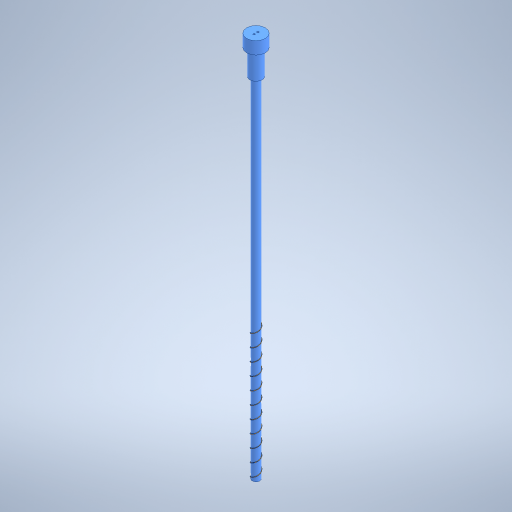
# Autodesk Inventor part: heater plug
Saved by Autodesk Inventor 2023 (Build 270158030, 158C)
## iProperties
Created: 2025-06-04
Part Number: heater plug
Material: Generisch
Document SubType Name: Modeling
Designer: Julian
Density: 1 g/cm^3
Appearance: Vorgabe
Author: Julian
Autodesk Inventor part; units mm, degrees
ref_plane "YZ Plane" through (0, 0, 0) normal (1, 0, 0) x (0, 1, 0)
ref_plane "XZ Plane" through (0, 0, 0) normal (0, 1, 0) x (-1, 0, 0)
sketch "Skizze1" plane through (0, 0, 0) normal (0, 1, 0) x (-1, 0, 0)
  circle A0 centre (0, 0) radius 7.5
  circle A1 centre (0, 0) radius 5
  circle A2 centre (0, 0) radius 3
  line L0 (0, 5) -> (0, 1.5)
  line L1 (0, 1.5) -> (0, -1.5)
  circle A3 centre (0, -1.5) radius 0.75
  circle A4 centre (0, 1.5) radius 0.75
  dimension "d1" = 10
  dimension "d0" = 15
  dimension "d2" = 6
  dimension "d3" = 3.5
  dimension "d4" = 3
  dimension "d5" = 1.5
  dimension "d6" = 1.5
  constraints: 5 coincident, 4 centre point, 4 end point, 1 point on line, 1 vertical, 1 vertical alignment, 2 other
  measures "d0" diameter of A0
  measures "d2" diameter of A2
  measures "d3" distance of L0.start L0.end
  measures "d4" distance of L0.end L1.end
  measures "d5" diameter of A3
  measures "d6" diameter of A4
extrude "Extrusion1" add sketch "Skizze1" along normal blind 10 contours A0 | A2 | A1
extrude "Extrusion2" add sketch "Skizze1" against normal blind 20 contours A2 | A1
extrude "Extrusion3" add sketch "Skizze1" against normal blind 300 contours A2
ref_plane "Arbeitsebene1" through (0, -190, 0) normal (0, 1, 0) x (1, 0, 0)
sketch "Skizze2" plane through (0, -190, 0) normal (0, 1, 0) x (1, 0, 0)
  circle A0 centre (0, 0) radius 3 projected
  line L0 (-3, 0) -> (-3.4, 0)
  line L1 (-3.4, 0) -> (-3.4, 1)
  line L2 (-3.4, 1) -> (-3, 1)
  line L3 (-3, 1) -> (-3, 0)
  dimension "d16" = 0.4
  dimension "d17" = 1
  constraints: 8 end point, 2 parallel, 1 horizontal, 1 horizontal alignment, 1 perpendicular, 1 other
  measures "d16" distance of L1.end L2.end
  measures "d17" distance of L0.end L1.end
coil "Spirale1" sketch "Skizze2" operation add axis through (0, 0, 0) along (0, -1, 0) pitch 10 turns 11 hand right contours L0 L1 L2 L3
